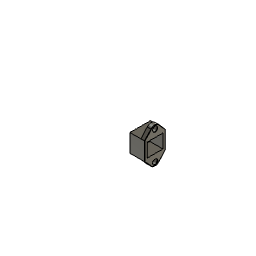
Motor Mount (Autodesk Fusion 360 design; units mm, degrees)
Autodesk Fusion 360 part; units mm, degrees
sketch "Sketch1" plane through (0, 0, 0) normal (-1, 0, 0) x (0, -1, 0)
  circle A0 centre (-15, 24.65) radius 1.4
  circle A1 centre (-87, 27) radius 1.75
  circle A2 centre (-3, 27) radius 1.75
  circle A3 centre (-15, 2.85) radius 1.4
  circle A4 centre (-15, 13.75) radius 2.5
  circle A5 centre (-75, 13.75) radius 1.75
  line L0 (0, 0) -> (0, 30)
  line L1 (0, 30) -> (-90, 30)
  line L2 (-90, 30) -> (-90, 0)
  line L3 (-90, 0) -> (0, 0)
  line L4 (-7.1, 20.65) -> (-22.9, 20.65)
  line L5 (-22.9, 20.65) -> (-22.9, 6.85)
  line L6 (-22.9, 6.85) -> (-7.1, 6.85)
  line L7 (-7.1, 6.85) -> (-7.1, 20.65)
  line L8 (-7.1, 20.65) -> (-22.9, 6.85) construction
  line L9 (-22.9, 20.65) -> (-7.1, 6.85) construction
  circle A6 centre (-15, 24.65) radius 1.75
  circle A7 centre (-15, 2.85) radius 1.75
  circle A8 centre (-15, 13.75) radius 6
  line L10 (-17.8125, 19.05) -> (-12.1875, 19.05)
  line L11 (-17.8125, 8.45) -> (-12.1875, 8.45)
  line L12 (-9, 8.75) -> (-21, 18.75) construction
  line L13 (-21, 8.75) -> (-9, 18.75) construction
  line L14 (-21, 19.05) -> (-9, 19.05)
  line L15 (-9, 19.05) -> (-9, 8.45)
  line L16 (-9, 8.45) -> (-21, 8.45)
  line L17 (-21, 8.45) -> (-21, 19.05)
  line L18 (-15, 2.85) -> (-15, 0) construction
  line L19 (-15, 0) -> (-16.75, 0) construction
  line L20 (-16.75, 0) -> (-13.25, 0) construction
  line L21 (-22.9, 6.85) -> (-16.75, 0)
  line L22 (-13.25, 0) -> (-7.1, 6.85)
  line L23 (-15, 24.65) -> (-15, 27.5) construction
  line L24 (-15, 27.5) -> (-13.25, 27.5) construction
  line L25 (-13.25, 27.5) -> (-16.75, 27.5) construction
  line L26 (-16.75, 27.5) -> (-22.9, 20.65)
  line L27 (-16.75, 27.5) -> (-13.25, 27.5)
  line L28 (-13.25, 27.5) -> (-7.1, 20.65)
  line L29 (-16.75, 0) -> (-15, -1.9492)
  line L30 (-15, -1.9492) -> (-13.25, 0)
  line L31 (-16.75, 27.5) -> (-15, 29.4492)
  line L32 (-13.25, 27.5) -> (-15, 29.4492)
  point P0 (-15, 13.75)
  point P1 (-15, 13.75)
  dimension "d76" = 15.8
  dimension "d77" = 13.8
  dimension "d78" = 3.5
  dimension "d79" = 3.5
  dimension "d86" = 12
  dimension "d87" = 5.3
  dimension "d88" = 5.3
  dimension "d91" = 12
  dimension "d92" = 10.6
  dimension "d93" = 5.3
  dimension "d94" = 6
  dimension "d104" = 1.75
  dimension "d105" = 3.5
  dimension "d106" = 2.85
  dimension "d107" = 2.85
  dimension "d108" = 1.75
  dimension "d109" = 3.5
  constraint horizontal L4
  constraint perpendicular L4 L5
  constraint parallel L4 L6
  constraint parallel L5 L7
  constraint coincident L8 P1
  constraint coincident L9 P1
  constraint coincident P1 P0
  constraint concentric A0 A6
  constraint concentric A3 A7
  constraint concentric A4 A8
  constraint coincident A8 L10.start
  constraint coincident A8 L10.end
  constraint horizontal L10
  constraint coincident A8 L11.start
  constraint coincident A8 L11.end
  constraint parallel L10 L11
  constraint coincident L12 P1
  constraint coincident L13 P1
  constraint horizontal L14
  constraint vertical L15
  constraint horizontal L16
  constraint vertical L17
  constraint coincident A3.centre A7.centre
  constraint coincident L3 L18.end
  constraint perpendicular L3 L18
  constraint perpendicular L18 L19
  constraint perpendicular L18 L20
  constraint coincident A0.centre A6.centre
  constraint vertical L23
  constraint perpendicular L23 L24
  constraint parallel L24 L25
  constraint parallel L21 L29
  constraint parallel L22 L30
  constraint parallel L26 L31
  measures "d76" distance of L5.end L6.end
  measures "d77" distance of L4.end L5.end
  measures "d78" diameter of A6
  measures "d79" diameter of A7
  measures "d86" diameter of A8
  measures "d87" distance of P1 L10
  measures "d88" distance of P1 L11
  measures "d91" distance of L14.start L14.end
  measures "d92" distance of L14.start L16.end
  measures "d93" distance of P1 L14
  measures "d94" distance of P1 L17
  measures "d104" distance of L18.end L19.end
  measures "d105" distance of L19.end L20.end
  measures "d106" distance of A3.centre L18.end
  measures "d107" distance of A0.centre L23.end
  measures "d108" distance of L23.end L24.end
  measures "d109" distance of L24.end L25.end
extrude "Extrude1" add sketch "Sketch1" along normal blind 3 contours L3 L29 L30 | L3 L6 L21 L22 | L4 L5 L6 L7 | L4 L26 L27 L28 | L27 L31 L32 | A8 L10 L11 L14 L16 | A8 L15 L16 | A8 L14 L15 | A8 L10 L14 | A8 L11 L16 | A8 L14 L17 | A8 L16 L17
extrude "Extrude2" cut sketch "Sketch1" along normal blind 3 contours A8 L10 L11 L14 L16 | A8 L15 L16 | A8 L14 L15 | A8 L14 L17 | A8 L16 L17
extrude "Extrude3" add sketch "Sketch1" along normal blind 11.6 contours L4 L5 L6 L7 | A8 L10 L14 | A8 L11 L16
extrude "Extrude4" add sketch "Sketch1" against normal blind 1.6 from surface at 11.6 contours A8 L15 L16 | A8 L14 L15 | A8 L14 L17 | A8 L16 L17
fillet "Fillet1" radius 4 2 edges at (-1.5, 15, 29.4492) (-1.5, 15, -1.9492)
chamfer "Chamfer1" distance 0.2 angle 45 18 edges at (-11.6, 7.1, 13.75) (-11.6, 15, 20.65) (-11.6, 22.9, 13.75) (-11.6, 15, 6.85) (0, 7.1, 13.75) (0, 9.5618, 23.392) (0, 15, 27.4617) (0, 20.4382, 23.392) (0, 9.5618, 4.108) (0, 15, 0.0383) (0, 20.4382, 4.108) (0, 22.9, 13.75) (0, 16.6316, 25.2828) (0, 16.6316, 3.4828) (-10, 20.1417, 10.6577) (-10, 20.1417, 16.8423) (-10, 9.8583, 16.8423) (-10, 9.8583, 10.6577)
chamfer "Chamfer1" distance 0.2 angle 45 2 edges at (-3, 15, 20.65) (-3, 15, 6.85)
